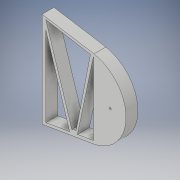
# Autodesk Inventor part: Radaufhängung
Saved by Autodesk Inventor 2017 (Build 210142000, 142)
## iProperties
Part Number: Radaufhängung
Material: Generisch
Document SubType Name: Modeling
Designer: chris
Density: 1 g/cm^3
Appearance: Vorgabe
Author: chris
Autodesk Inventor part; units mm, degrees
ref_plane "YZ Plane" through (0, 0, 0) normal (1, 0, 0) x (0, 1, 0)
ref_plane "XZ Plane" through (0, 0, 0) normal (0, 1, 0) x (-1, 0, 0)
ref_plane "XY Plane" through (0, 0, 0) normal (0, 0, 1) x (1, 0, 0)
sketch "Skizze1" plane through (0, 0, 0) normal (0, 1, 0) x (-1, 0, 0)
  line L0 (60.2262, 75.3938) -> (60.2262, -74.6062)
  line L1 (60.2262, -74.6062) -> (-19.7738, -60.5)
  line L2 (-19.7738, -60.5) -> (-19.7738, 61.2877)
  line L3 (-19.7738, 61.2877) -> (60.2262, 75.3938)
  arc A0 (-19.7738, 61.2877) -> (-19.7738, -60.5) centre (-8.1145, 0.3938) ccw
  circle A1 centre (-48.1145, 0) radius 1.7
  line L4 (60.2262, 60.3938) -> (20.2262, -67.5531)
  line L5 (7.0615, -65.2318) -> (-19.7534, 61.2913)
  line L6 (60.2262, 75.3938) -> (16.5507, -62.5531)
  line L7 (16.5507, -62.5531) -> (9.219, -60.2318)
  line L8 (9.219, -60.2318) -> (-14.7534, 62.1729)
  line L9 (66.5322, 80) -> (66.5322, -80)
  line L10 (66.5322, -80) -> (-19.7534, -65.5678)
  line L11 (66.5322, 80) -> (-20.7513, 65.9995)
  arc A2 (-20.7513, 65.9995) -> (-19.7534, -65.5678) centre (-7.5537, 0.3121) ccw
  point P0 (0, 0)
  point P1 (0, 0)
  dimension "d6" = 150
  dimension "d8" = 80
  dimension "d9" = 100
  dimension "d10" = 100
  dimension "d12" = 60.5
  dimension "d15" = 62
  dimension "d16" = 3.4
  dimension "d17" = 40
  dimension "d18" = 15
  dimension "d22" = 5
  dimension "d23" = 5
  dimension "d25" = 5
  dimension "d26" = 5
  dimension "d27" = 3.1473
  dimension "d28" = 7.3316
  dimension "d29" = 160
  dimension "d30" = 80
  dimension "d31" = 67
  constraints: 24 end point, 5 point on circle, 5 point on line, 3 centre point, 2 vertical, 1 coincident, 1 midpoint, 1 parallel, 1 perpendicular
  measures "d6" distance of L0.start L0.end
  measures "d8" distance between parallel lines of L0 L2
  measures "d9" angle of L2 L3
  measures "d10" angle of L2 L1
  measures "d12" vertical distance of point (0, 0) L1.end
  measures "d15" radius of A0
  measures "d16" diameter of A1
  measures "d17" horizontal distance of A1.centre A0.centre
  measures "d18" distance of L4.start L0.start
  measures "d22" vertical distance of L4.end L6.end
  measures "d23" vertical distance of L5.start L7.end
  measures "d25" horizontal distance of L8.end L5.end
  measures "d26" distance from line of L4 L6.end
  measures "d27" distance from line of L5 L7.end
  measures "d28" horizontal distance of L6.end L7.end
  measures "d29" distance of L9.start L9.end
  measures "d30" vertical distance of point (0, 0) L9.start
  measures "d31" radius of A2
extrude "Extrusion1" add sketch "Skizze1" along normal blind 20 contours L0 L4 L1 L5 L3 L8 L7 L6 | L2 A0 | L9 L10 A2 L11
